Autodesk Fusion 360 part; units mm, degrees
(part 2 of 3)
  spline S21 degree 5 poles (-5.7507, 8.7852) (-5.7508, 8.7791) (-5.7509, 8.7671) (-5.7511, 8.7491) (-5.7512, 8.7251) (-5.7512, 8.6951) (-5.751, 8.6652) (-5.7507, 8.6353) (-5.7502, 8.6055) (-5.7495, 8.5758) (-5.7487, 8.5461) (-5.7478, 8.5165) (-5.7467, 8.4869) (-5.7454, 8.4574) (-5.7439, 8.428) (-5.7423, 8.3986) (-5.7406, 8.3693) (-5.7387, 8.34) (-5.7366, 8.3109) (-5.7343, 8.2817) (-5.7319, 8.2527) (-5.7293, 8.2237) (-5.7266, 8.1948) (-5.7237, 8.166) (-5.7206, 8.1372) (-5.7174, 8.1086) (-5.714, 8.0799) (-5.7104, 8.0514) (-5.7067, 8.023) (-5.7027, 7.9946) (-5.6987, 7.9663) (-5.6944, 7.9381) (-5.69, 7.91) (-5.6854, 7.8819) (-5.6806, 7.854) (-5.6756, 7.8261) (-5.6705, 7.7983) (-5.6652, 7.7706) (-5.6597, 7.743) (-5.654, 7.7156) (-5.6482, 7.6882) (-5.6421, 7.6609) (-5.6359, 7.6337) (-5.6295, 7.6066) (-5.6228, 7.5796) (-5.616, 7.5527) (-5.609, 7.5259) (-5.6019, 7.4993) (-5.5945, 7.4727) (-5.5869, 7.4463) (-5.5791, 7.42) (-5.5711, 7.3938) (-5.5629, 7.3677) (-5.5544, 7.3418) (-5.5457, 7.316) (-5.5368, 7.2904) (-5.5277, 7.2649) (-5.5184, 7.2395) (-5.5089, 7.2142) (-5.4992, 7.1891) (-5.4892, 7.1642) (-5.4788, 7.1395) (-5.4681, 7.115) (-5.4571, 7.0908) (-5.4457, 7.0667) (-5.4342, 7.0428) (-5.4224, 7.0191) (-5.4105, 6.9954) (-5.3984, 6.972) (-5.3859, 6.9488) (-5.3726, 6.9261) (-5.3612, 6.9086) (-5.3521, 6.8957) (-5.3458, 6.8874) (-5.3426, 6.8832) knots -1 -1 -1 -1 -1 -1 -0.98571429 -0.97142857 -0.95714286 -0.94285714 -0.92857143 -0.91428571 -0.9 -0.88571429 -0.87142857 -0.85714286 -0.84285714 -0.82857143 -0.81428571 -0.8 -0.78571429 -0.77142857 -0.75714286 -0.74285714 -0.72857143 -0.71428571 -0.7 -0.68571429 -0.67142857 -0.65714286 -0.64285714 -0.62857143 -0.61428571 -0.6 -0.58571429 -0.57142857 -0.55714286 -0.54285714 -0.52857143 -0.51428571 -0.5 -0.48571429 -0.47142857 -0.45714286 -0.44285714 -0.42857143 -0.41428571 -0.4 -0.38571429 -0.37142857 -0.35714286 -0.34285714 -0.32857143 -0.31428571 -0.3 -0.28571429 -0.27142857 -0.25714286 -0.24285714 -0.22857143 -0.21428571 -0.2 -0.18571429 -0.17142857 -0.15714286 -0.14285714 -0.12857143 -0.11428571 -0.1 -0.08571429 -0.07142857 -0.05714286 -0.04285714 -0.02857143 -0.01428571 0 0 0 0 0 0
  line L21 (-5.3426, 6.8832) -> (-4.7509, 6.121)
  arc A42 (-4.8145, 5.44) -> (-4.7509, 6.121) centre (-5.1459, 5.8144) ccw
  arc A43 (-4.8145, 5.44) -> (-5.44, 4.8145) centre (0, 0) ccw
  arc A44 (-6.121, 4.7509) -> (-5.44, 4.8145) centre (-5.8144, 5.1459) ccw
  line L22 (-6.121, 4.7509) -> (-6.8832, 5.3426)
  spline S22 degree 5 poles (-6.8832, 5.3426) (-6.8874, 5.3458) (-6.8957, 5.3521) (-6.9086, 5.3612) (-6.9261, 5.3726) (-6.9488, 5.3859) (-6.972, 5.3984) (-6.9954, 5.4105) (-7.0191, 5.4224) (-7.0428, 5.4342) (-7.0667, 5.4457) (-7.0908, 5.4571) (-7.115, 5.4681) (-7.1395, 5.4788) (-7.1642, 5.4892) (-7.1891, 5.4992) (-7.2142, 5.5089) (-7.2395, 5.5184) (-7.2649, 5.5277) (-7.2904, 5.5368) (-7.316, 5.5457) (-7.3418, 5.5544) (-7.3677, 5.5629) (-7.3938, 5.5711) (-7.42, 5.5791) (-7.4463, 5.5869) (-7.4727, 5.5945) (-7.4993, 5.6019) (-7.5259, 5.609) (-7.5527, 5.616) (-7.5796, 5.6228) (-7.6066, 5.6295) (-7.6337, 5.6359) (-7.6609, 5.6421) (-7.6882, 5.6482) (-7.7156, 5.654) (-7.743, 5.6597) (-7.7706, 5.6652) (-7.7983, 5.6705) (-7.8261, 5.6756) (-7.854, 5.6806) (-7.8819, 5.6854) (-7.91, 5.69) (-7.9381, 5.6944) (-7.9663, 5.6987) (-7.9946, 5.7027) (-8.023, 5.7067) (-8.0514, 5.7104) (-8.0799, 5.714) (-8.1086, 5.7174) (-8.1372, 5.7206) (-8.166, 5.7237) (-8.1948, 5.7266) (-8.2237, 5.7293) (-8.2527, 5.7319) (-8.2817, 5.7343) (-8.3109, 5.7366) (-8.34, 5.7387) (-8.3693, 5.7406) (-8.3986, 5.7423) (-8.428, 5.7439) (-8.4574, 5.7454) (-8.4869, 5.7467) (-8.5165, 5.7478) (-8.5461, 5.7487) (-8.5758, 5.7495) (-8.6055, 5.7502) (-8.6353, 5.7507) (-8.6652, 5.751) (-8.6951, 5.7512) (-8.7251, 5.7512) (-8.7491, 5.7511) (-8.7671, 5.7509) (-8.7791, 5.7508) (-8.7852, 5.7507) knots 0 0 0 0 0 0 0.01428571 0.02857143 0.04285714 0.05714286 0.07142857 0.08571429 0.1 0.11428571 0.12857143 0.14285714 0.15714286 0.17142857 0.18571429 0.2 0.21428571 0.22857143 0.24285714 0.25714286 0.27142857 0.28571429 0.3 0.31428571 0.32857143 0.34285714 0.35714286 0.37142857 0.38571429 0.4 0.41428571 0.42857143 0.44285714 0.45714286 0.47142857 0.48571429 0.5 0.51428571 0.52857143 0.54285714 0.55714286 0.57142857 0.58571429 0.6 0.61428571 0.62857143 0.64285714 0.65714286 0.67142857 0.68571429 0.7 0.71428571 0.72857143 0.74285714 0.75714286 0.77142857 0.78571429 0.8 0.81428571 0.82857143 0.84285714 0.85714286 0.87142857 0.88571429 0.9 0.91428571 0.92857143 0.94285714 0.95714286 0.97142857 0.98571429 1 1 1 1 1 1
  arc A45 (-8.7852, 5.7507) -> (-9.3729, 4.7328) centre (0, 0) ccw
  spline S23 degree 5 poles (-9.3729, 4.7328) (-9.3699, 4.7276) (-9.364, 4.7171) (-9.3551, 4.7014) (-9.3432, 4.6805) (-9.3282, 4.6546) (-9.3131, 4.6288) (-9.2979, 4.6031) (-9.2826, 4.5775) (-9.2671, 4.5521) (-9.2516, 4.5268) (-9.236, 4.5016) (-9.2202, 4.4766) (-9.2044, 4.4516) (-9.1884, 4.4269) (-9.1723, 4.4022) (-9.1561, 4.3777) (-9.1398, 4.3534) (-9.1234, 4.3291) (-9.1069, 4.305) (-9.0903, 4.2811) (-9.0736, 4.2573) (-9.0568, 4.2336) (-9.0399, 4.2101) (-9.0228, 4.1867) (-9.0057, 4.1635) (-8.9884, 4.1404) (-8.9711, 4.1175) (-8.9536, 4.0948) (-8.936, 4.0721) (-8.9183, 4.0497) (-8.9005, 4.0274) (-8.8826, 4.0052) (-8.8646, 3.9833) (-8.8465, 3.9614) (-8.8283, 3.9398) (-8.8099, 3.9183) (-8.7915, 3.897) (-8.773, 3.8758) (-8.7543, 3.8549) (-8.7355, 3.8341) (-8.7166, 3.8134) (-8.6976, 3.793) (-8.6785, 3.7728) (-8.6593, 3.7527) (-8.64, 3.7328) (-8.6205, 3.7131) (-8.601, 3.6936) (-8.5813, 3.6743) (-8.5615, 3.6552) (-8.5416, 3.6363) (-8.5216, 3.6176) (-8.5014, 3.5992) (-8.4812, 3.581) (-8.4608, 3.563) (-8.4402, 3.5453) (-8.4196, 3.5277) (-8.3989, 3.5104) (-8.378, 3.4932) (-8.357, 3.4764) (-8.3359, 3.4598) (-8.3146, 3.4436) (-8.293, 3.4277) (-8.2714, 3.4122) (-8.2495, 3.3971) (-8.2275, 3.3822) (-8.2055, 3.3675) (-8.1834, 3.3529) (-8.1611, 3.3387) (-8.1387, 3.3249) (-8.1159, 3.3119) (-8.0972, 3.3024) (-8.0829, 3.2958) (-8.0733, 3.2917) (-8.0684, 3.2898) knots -1 -1 -1 -1 -1 -1 -0.98571429 -0.97142857 -0.95714286 -0.94285714 -0.92857143 -0.91428571 -0.9 -0.88571429 -0.87142857 -0.85714286 -0.84285714 -0.82857143 -0.81428571 -0.8 -0.78571429 -0.77142857 -0.75714286 -0.74285714 -0.72857143 -0.71428571 -0.7 -0.68571429 -0.67142857 -0.65714286 -0.64285714 -0.62857143 -0.61428571 -0.6 -0.58571429 -0.57142857 -0.55714286 -0.54285714 -0.52857143 -0.51428571 -0.5 -0.48571429 -0.47142857 -0.45714286 -0.44285714 -0.42857143 -0.41428571 -0.4 -0.38571429 -0.37142857 -0.35714286 -0.34285714 -0.32857143 -0.31428571 -0.3 -0.28571429 -0.27142857 -0.25714286 -0.24285714 -0.22857143 -0.21428571 -0.2 -0.18571429 -0.17142857 -0.15714286 -0.14285714 -0.12857143 -0.11428571 -0.1 -0.08571429 -0.07142857 -0.05714286 -0.04285714 -0.02857143 -0.01428571 0 0 0 0 0 0
  line L23 (-8.0684, 3.2898) -> (-7.1749, 2.9254)
  arc A46 (-6.8895, 2.3039) -> (-7.1749, 2.9254) centre (-7.3637, 2.4624) ccw
  arc A47 (-6.8895, 2.3039) -> (-7.1184, 1.4495) centre (0, 0) ccw
  circle A48 centre (0, 0) radius 1.25
  line L24 (-9.0903, -5.085) -> (-5.33, 8.9489)
  arc A49 (-2.722, 8.2501) -> (-5.33, 8.9489) centre (-4.026, 8.5995) ccw
  line L25 (-2.722, 8.2501) -> (-6.4823, -5.7838)
  arc A50 (-9.0903, -5.085) -> (-6.4823, -5.7838) centre (-7.7863, -5.4344) ccw
  line L26 (-7.7981, 1.2832) -> (-9.4767, -4.9815)
  arc A51 (-9.4767, -4.9815) -> (-6.096, -5.8874) centre (-7.7863, -5.4344) ccw
  line L27 (-6.096, -5.8874) -> (-2.3356, 8.1466)
  arc A52 (-2.3356, 8.1466) -> (-5.7163, 9.0525) centre (-4.026, 8.5995) ccw
  line L28 (-5.7163, 9.0525) -> (-7.2804, 3.2151)
  line L29 (-7.2804, 3.2151) -> (-36.2582, 10.9797)
  line L30 (-36.2582, 10.9797) -> (-36.7759, 9.0478)
  line L31 (-36.7759, 9.0478) -> (-7.7981, 1.2832)
  circle A53 centre (-5.8457, 1.7953) radius 1.15
extrude "Extrude1" add sketch "sketch 238" along normal blind 2 contours A0 L0 S23 L23 A46 L24 L26 L29 L30 L31 | A0 L0 L1 L24 L26 | L1 S2 A5 L3 A6 L24 L25 A50 L26 A51 L27 | L22 S23 L23 A46 L24 L28 L29 | S2 A5 L24 A50 | A40 L20 A41 S21 L22 L24 A49 L25 L27 A52 L28 | A41 S21 L24 A49 | L3 A6 A40 L20 L25 L27
sketch "Sketch1" plane through (0, 0, 5) normal (0, 0, 1) x (-1, 0, 0)
  arc A0 (-2.722, 8.2501) -> (-5.33, 8.9489) centre (-4.026, 8.5995) ccw
  line L0 (-2.722, 8.2501) -> (-6.4823, -5.7838)
  arc A1 (-9.0903, -5.085) -> (-6.4823, -5.7838) centre (-7.7863, -5.4344) ccw
  line L1 (-9.0903, -5.085) -> (-5.33, 8.9489)
  line L2 (-36.7759, 9.0478) -> (-7.7981, 1.2832)
  line L3 (-7.7981, 1.2832) -> (-9.4767, -4.9815)
  arc A2 (-9.4767, -4.9815) -> (-6.096, -5.8874) centre (-7.7863, -5.4344) ccw
  line L4 (-6.096, -5.8874) -> (-2.3356, 8.1466)
  arc A3 (-2.3356, 8.1466) -> (-5.7163, 9.0525) centre (-4.026, 8.5995) ccw
  line L5 (-5.7163, 9.0525) -> (-7.2804, 3.2151)
  line L6 (-7.2804, 3.2151) -> (-36.2582, 10.9797)
  line L7 (-36.2582, 10.9797) -> (-36.7759, 9.0478)
  line L8 (-4.6022, 1.2331) -> (-7.2102, 1.932)
  line L9 (-7.2102, 1.932) -> (-7.214, 1.933)
  line L10 (-6.9513, 2.8979) -> (-36.2582, 10.9797)
  line L11 (-7.2804, 3.2151) -> (-6.8941, 3.1116)
  line L12 (-6.8941, 3.1116) -> (-7.476, 0.9679)
  line L13 (-7.8546, 1.0723) -> (-7.2804, 3.2151)
  line L14 (-7.2804, 3.2151) -> (-36.2582, 10.9797)
  line L15 (-36.2582, 10.9797) -> (-36.7759, 9.0478)
  line L16 (-7.7981, 1.2832) -> (-36.7759, 9.0478)
  line L17 (-7.8546, 1.0723) -> (-36.7759, 9.0478)
  point P0 (-7.3369, 3.0042)
  constraint midpoint L0 L8.start
  constraint midpoint L1 L8.end
  constraint coincident L1 L10.start
  constraint coincident L5.end L6.start
  constraint coincident L1 L11.end
  constraint perpendicular L1 L11
  constraint coincident L3 L13.start
  constraint coincident L6.end L7.start
  constraint coincident L2.start L7.end
  constraint coincident L2.end L3.start
  constraint coincident L13 P0
  constraint coincident L10 P0
extrude "Extrude2" cut sketch "Sketch1" against normal blind 9.5 contours L6 L10 L13 L14
extrude "Extrude3" add sketch "Sketch1" against normal blind 2 contours L2 L3 L13 L16 L17

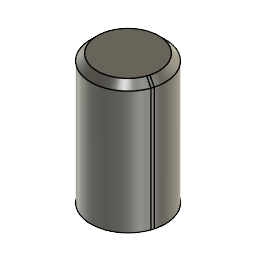
design "MiniKey_GearPin"
Autodesk Fusion 360 part; units mm, degrees
other "Sketch1"
sketch "sketch 232" plane through (0, 0, 3) normal (0, 0, 1) x (-1, 0, 0)
  arc A0 (-7.6764, 1.0539) -> (-7.1184, 1.4495) centre (-7.6084, 1.5493) ccw
  line L0 (-7.6764, 1.0539) -> (-8.6323, 1.1852)
  spline S0 degree 5 poles (-8.6323, 1.1852) (-8.6375, 1.1859) (-8.6479, 1.1872) (-8.6636, 1.1886) (-8.6845, 1.1897) (-8.7108, 1.1899) (-8.7371, 1.1892) (-8.7635, 1.188) (-8.7899, 1.1864) (-8.8164, 1.1847) (-8.8428, 1.1828) (-8.8693, 1.1806) (-8.8958, 1.178) (-8.9224, 1.1751) (-8.949, 1.1717) (-8.9756, 1.1679) (-9.0022, 1.1638) (-9.0288, 1.1594) (-9.0554, 1.1547) (-9.0821, 1.1498) (-9.1087, 1.1447) (-9.1354, 1.1393) (-9.1621, 1.1337) (-9.1887, 1.1278) (-9.2154, 1.1217) (-9.2421, 1.1153) (-9.2688, 1.1086) (-9.2955, 1.1017) (-9.3222, 1.0946) (-9.3488, 1.0873) (-9.3755, 1.0797) (-9.4022, 1.072) (-9.4289, 1.064) (-9.4555, 1.0558) (-9.4822, 1.0474) (-9.5089, 1.0387) (-9.5355, 1.0299) (-9.5622, 1.0209) (-9.5888, 1.0116) (-9.6154, 1.0022) (-9.642, 0.9925) (-9.6686, 0.9827) (-9.6952, 0.9727) (-9.7218, 0.9624) (-9.7483, 0.952) (-9.7749, 0.9414) (-9.8014, 0.9306) (-9.8279, 0.9196) (-9.8544, 0.9085) (-9.8809, 0.8971) (-9.9074, 0.8856) (-9.9338, 0.8739) (-9.9602, 0.862) (-9.9866, 0.8499) (-10.013, 0.8376) (-10.0394, 0.8252) (-10.0657, 0.8126) (-10.092, 0.7998) (-10.1183, 0.7868) (-10.1446, 0.7737) (-10.1708, 0.7604) (-10.197, 0.7469) (-10.2232, 0.7333) (-10.2494, 0.7195) (-10.2755, 0.7055) (-10.3016, 0.6914) (-10.3277, 0.677) (-10.3538, 0.6626) (-10.3798, 0.6479) (-10.4058, 0.6331) (-10.4317, 0.6182) (-10.4525, 0.6061) (-10.468, 0.5969) (-10.4784, 0.5908) (-10.4835, 0.5877) knots 0 0 0 0 0 0 0.01428571 0.02857143 0.04285714 0.05714286 0.07142857 0.08571429 0.1 0.11428571 0.12857143 0.14285714 0.15714286 0.17142857 0.18571429 0.2 0.21428571 0.22857143 0.24285714 0.25714286 0.27142857 0.28571429 0.3 0.31428571 0.32857143 0.34285714 0.35714286 0.37142857 0.38571429 0.4 0.41428571 0.42857143 0.44285714 0.45714286 0.47142857 0.48571429 0.5 0.51428571 0.52857143 0.54285714 0.55714286 0.57142857 0.58571429 0.6 0.61428571 0.62857143 0.64285714 0.65714286 0.67142857 0.68571429 0.7 0.71428571 0.72857143 0.74285714 0.75714286 0.77142857 0.78571429 0.8 0.81428571 0.82857143 0.84285714 0.85714286 0.87142857 0.88571429 0.9 0.91428571 0.92857143 0.94285714 0.95714286 0.97142857 0.98571429 1 1 1 1 1 1
  arc A1 (-10.4835, 0.5877) -> (-10.4835, -0.5877) centre (0, 0) ccw
  spline S1 degree 5 poles (-10.4835, -0.5877) (-10.4784, -0.5908) (-10.468, -0.5969) (-10.4525, -0.6061) (-10.4317, -0.6182) (-10.4058, -0.6331) (-10.3798, -0.6479) (-10.3538, -0.6626) (-10.3277, -0.677) (-10.3016, -0.6914) (-10.2755, -0.7055) (-10.2494, -0.7195) (-10.2232, -0.7333) (-10.197, -0.7469) (-10.1708, -0.7604) (-10.1446, -0.7737) (-10.1183, -0.7868) (-10.092, -0.7998) (-10.0657, -0.8126) (-10.0394, -0.8252) (-10.013, -0.8376) (-9.9866, -0.8499) (-9.9602, -0.862) (-9.9338, -0.8739) (-9.9074, -0.8856) (-9.8809, -0.8971) (-9.8544, -0.9085) (-9.8279, -0.9196) (-9.8014, -0.9306) (-9.7749, -0.9414) (-9.7483, -0.952) (-9.7218, -0.9624) (-9.6952, -0.9727) (-9.6686, -0.9827) (-9.642, -0.9925) (-9.6154, -1.0022) (-9.5888, -1.0116) (-9.5622, -1.0209) (-9.5355, -1.0299) (-9.5089, -1.0387) (-9.4822, -1.0474) (-9.4555, -1.0558) (-9.4289, -1.064) (-9.4022, -1.072) (-9.3755, -1.0797) (-9.3488, -1.0873) (-9.3222, -1.0946) (-9.2955, -1.1017) (-9.2688, -1.1086) (-9.2421, -1.1153) (-9.2154, -1.1217) (-9.1887, -1.1278) (-9.1621, -1.1337) (-9.1354, -1.1393) (-9.1087, -1.1447) (-9.0821, -1.1498) (-9.0554, -1.1547) (-9.0288, -1.1594) (-9.0022, -1.1638) (-8.9756, -1.1679) (-8.949, -1.1717) (-8.9224, -1.1751) (-8.8958, -1.178) (-8.8693, -1.1806) (-8.8428, -1.1828) (-8.8164, -1.1847) (-8.7899, -1.1864) (-8.7635, -1.188) (-8.7371, -1.1892) (-8.7108, -1.1899) (-8.6845, -1.1897) (-8.6636, -1.1886) (-8.6479, -1.1872) (-8.6375, -1.1859) (-8.6323, -1.1852) knots -1 -1 -1 -1 -1 -1 -0.98571429 -0.97142857 -0.95714286 -0.94285714 -0.92857143 -0.91428571 -0.9 -0.88571429 -0.87142857 -0.85714286 -0.84285714 -0.82857143 -0.81428571 -0.8 -0.78571429 -0.77142857 -0.75714286 -0.74285714 -0.72857143 -0.71428571 -0.7 -0.68571429 -0.67142857 -0.65714286 -0.64285714 -0.62857143 -0.61428571 -0.6 -0.58571429 -0.57142857 -0.55714286 -0.54285714 -0.52857143 -0.51428571 -0.5 -0.48571429 -0.47142857 -0.45714286 -0.44285714 -0.42857143 -0.41428571 -0.4 -0.38571429 -0.37142857 -0.35714286 -0.34285714 -0.32857143 -0.31428571 -0.3 -0.28571429 -0.27142857 -0.25714286 -0.24285714 -0.22857143 -0.21428571 -0.2 -0.18571429 -0.17142857 -0.15714286 -0.14285714 -0.12857143 -0.11428571 -0.1 -0.08571429 -0.07142857 -0.05714286 -0.04285714 -0.02857143 -0.01428571 0 0 0 0 0 0
  line L1 (-8.6323, -1.1852) -> (-7.6764, -1.0539)
  arc A2 (-7.1184, -1.4495) -> (-7.6764, -1.0539) centre (-7.6084, -1.5493) ccw
  arc A3 (-7.1184, -1.4495) -> (-6.8895, -2.3039) centre (0, 0) ccw
  arc A4 (-7.1749, -2.9254) -> (-6.8895, -2.3039) centre (-7.3637, -2.4624) ccw
  line L2 (-7.1749, -2.9254) -> (-8.0684, -3.2898)
  spline S2 degree 5 poles (-8.0684, -3.2898) (-8.0733, -3.2917) (-8.0829, -3.2958) (-8.0972, -3.3024) (-8.1159, -3.3119) (-8.1387, -3.3249) (-8.1611, -3.3387) (-8.1834, -3.3529) (-8.2055, -3.3675) (-8.2275, -3.3822) (-8.2495, -3.3971) (-8.2714, -3.4122) (-8.293, -3.4277) (-8.3146, -3.4436) (-8.3359, -3.4598) (-8.357, -3.4764) (-8.378, -3.4932) (-8.3989, -3.5104) (-8.4196, -3.5277) (-8.4402, -3.5453) (-8.4608, -3.563) (-8.4812, -3.581) (-8.5014, -3.5992) (-8.5216, -3.6176) (-8.5416, -3.6363) (-8.5615, -3.6552) (-8.5813, -3.6743) (-8.601, -3.6936) (-8.6205, -3.7131) (-8.64, -3.7328) (-8.6593, -3.7527) (-8.6785, -3.7728) (-8.6976, -3.793) (-8.7166, -3.8134) (-8.7355, -3.8341) (-8.7543, -3.8549) (-8.773, -3.8758) (-8.7915, -3.897) (-8.8099, -3.9183) (-8.8283, -3.9398) (-8.8465, -3.9614) (-8.8646, -3.9833) (-8.8826, -4.0052) (-8.9005, -4.0274) (-8.9183, -4.0497) (-8.936, -4.0721) (-8.9536, -4.0948) (-8.9711, -4.1175) (-8.9884, -4.1404) (-9.0057, -4.1635) (-9.0228, -4.1867) (-9.0399, -4.2101) (-9.0568, -4.2336) (-9.0736, -4.2573) (-9.0903, -4.2811) (-9.1069, -4.305) (-9.1234, -4.3291) (-9.1398, -4.3534) (-9.1561, -4.3777) (-9.1723, -4.4022) (-9.1884, -4.4269) (-9.2044, -4.4516) (-9.2202, -4.4766) (-9.236, -4.5016) (-9.2516, -4.5268) (-9.2671, -4.5521) (-9.2826, -4.5775) (-9.2979, -4.6031) (-9.3131, -4.6288) (-9.3282, -4.6546) (-9.3432, -4.6805) (-9.3551, -4.7014) (-9.364, -4.7171) (-9.3699, -4.7276) (-9.3729, -4.7328) knots 0 0 0 0 0 0 0.01428571 0.02857143 0.04285714 0.05714286 0.07142857 0.08571429 0.1 0.11428571 0.12857143 0.14285714 0.15714286 0.17142857 0.18571429 0.2 0.21428571 0.22857143 0.24285714 0.25714286 0.27142857 0.28571429 0.3 0.31428571 0.32857143 0.34285714 0.35714286 0.37142857 0.38571429 0.4 0.41428571 0.42857143 0.44285714 0.45714286 0.47142857 0.48571429 0.5 0.51428571 0.52857143 0.54285714 0.55714286 0.57142857 0.58571429 0.6 0.61428571 0.62857143 0.64285714 0.65714286 0.67142857 0.68571429 0.7 0.71428571 0.72857143 0.74285714 0.75714286 0.77142857 0.78571429 0.8 0.81428571 0.82857143 0.84285714 0.85714286 0.87142857 0.88571429 0.9 0.91428571 0.92857143 0.94285714 0.95714286 0.97142857 0.98571429 1 1 1 1 1 1
  arc A5 (-9.3729, -4.7328) -> (-8.7852, -5.7507) centre (0, 0) ccw
  spline S3 degree 5 poles (-8.7852, -5.7507) (-8.7791, -5.7508) (-8.7671, -5.7509) (-8.7491, -5.7511) (-8.7251, -5.7512) (-8.6951, -5.7512) (-8.6652, -5.751) (-8.6353, -5.7507) (-8.6055, -5.7502) (-8.5758, -5.7495) (-8.5461, -5.7487) (-8.5165, -5.7478) (-8.4869, -5.7467) (-8.4574, -5.7454) (-8.428, -5.7439) (-8.3986, -5.7423) (-8.3693, -5.7406) (-8.34, -5.7387) (-8.3109, -5.7366) (-8.2817, -5.7343) (-8.2527, -5.7319) (-8.2237, -5.7293) (-8.1948, -5.7266) (-8.166, -5.7237) (-8.1372, -5.7206) (-8.1086, -5.7174) (-8.0799, -5.714) (-8.0514, -5.7104) (-8.023, -5.7067) (-7.9946, -5.7027) (-7.9663, -5.6987) (-7.9381, -5.6944) (-7.91, -5.69) (-7.8819, -5.6854) (-7.854, -5.6806) (-7.8261, -5.6756) (-7.7983, -5.6705) (-7.7706, -5.6652) (-7.743, -5.6597) (-7.7156, -5.654) (-7.6882, -5.6482) (-7.6609, -5.6421) (-7.6337, -5.6359) (-7.6066, -5.6295) (-7.5796, -5.6228) (-7.5527, -5.616) (-7.5259, -5.609) (-7.4993, -5.6019) (-7.4727, -5.5945) (-7.4463, -5.5869) (-7.42, -5.5791) (-7.3938, -5.5711) (-7.3677, -5.5629) (-7.3418, -5.5544) (-7.316, -5.5457) (-7.2904, -5.5368) (-7.2649, -5.5277) (-7.2395, -5.5184) (-7.2142, -5.5089) (-7.1891, -5.4992) (-7.1642, -5.4892) (-7.1395, -5.4788) (-7.115, -5.4681) (-7.0908, -5.4571) (-7.0667, -5.4457) (-7.0428, -5.4342) (-7.0191, -5.4224) (-6.9954, -5.4105) (-6.972, -5.3984) (-6.9488, -5.3859) (-6.9261, -5.3726) (-6.9086, -5.3612) (-6.8957, -5.3521) (-6.8874, -5.3458) (-6.8832, -5.3426) knots -1 -1 -1 -1 -1 -1 -0.98571429 -0.97142857 -0.95714286 -0.94285714 -0.92857143 -0.91428571 -0.9 -0.88571429 -0.87142857 -0.85714286 -0.84285714 -0.82857143 -0.81428571 -0.8 -0.78571429 -0.77142857 -0.75714286 -0.74285714 -0.72857143 -0.71428571 -0.7 -0.68571429 -0.67142857 -0.65714286 -0.64285714 -0.62857143 -0.61428571 -0.6 -0.58571429 -0.57142857 -0.55714286 -0.54285714 -0.52857143 -0.51428571 -0.5 -0.48571429 -0.47142857 -0.45714286 -0.44285714 -0.42857143 -0.41428571 -0.4 -0.38571429 -0.37142857 -0.35714286 -0.34285714 -0.32857143 -0.31428571 -0.3 -0.28571429 -0.27142857 -0.25714286 -0.24285714 -0.22857143 -0.21428571 -0.2 -0.18571429 -0.17142857 -0.15714286 -0.14285714 -0.12857143 -0.11428571 -0.1 -0.08571429 -0.07142857 -0.05714286 -0.04285714 -0.02857143 -0.01428571 0 0 0 0 0 0
  line L3 (-6.8832, -5.3426) -> (-6.121, -4.7509)
  arc A6 (-5.44, -4.8145) -> (-6.121, -4.7509) centre (-5.8144, -5.1459) ccw
  arc A7 (-5.44, -4.8145) -> (-4.8145, -5.44) centre (0, 0) ccw
  arc A8 (-4.7509, -6.121) -> (-4.8145, -5.44) centre (-5.1459, -5.8144) ccw
  line L4 (-4.7509, -6.121) -> (-5.3426, -6.8832)
  spline S4 degree 5 poles (-5.3426, -6.8832) (-5.3458, -6.8874) (-5.3521, -6.8957) (-5.3612, -6.9086) (-5.3726, -6.9261) (-5.3859, -6.9488) (-5.3984, -6.972) (-5.4105, -6.9954) (-5.4224, -7.0191) (-5.4342, -7.0428) (-5.4457, -7.0667) (-5.4571, -7.0908) (-5.4681, -7.115) (-5.4788, -7.1395) (-5.4892, -7.1642) (-5.4992, -7.1891) (-5.5089, -7.2142) (-5.5184, -7.2395) (-5.5277, -7.2649) (-5.5368, -7.2904) (-5.5457, -7.316) (-5.5544, -7.3418) (-5.5629, -7.3677) (-5.5711, -7.3938) (-5.5791, -7.42) (-5.5869, -7.4463) (-5.5945, -7.4727) (-5.6019, -7.4993) (-5.609, -7.5259) (-5.616, -7.5527) (-5.6228, -7.5796) (-5.6295, -7.6066) (-5.6359, -7.6337) (-5.6421, -7.6609) (-5.6482, -7.6882) (-5.654, -7.7156) (-5.6597, -7.743) (-5.6652, -7.7706) (-5.6705, -7.7983) (-5.6756, -7.8261) (-5.6806, -7.854) (-5.6854, -7.8819) (-5.69, -7.91) (-5.6944, -7.9381) (-5.6987, -7.9663) (-5.7027, -7.9946) (-5.7067, -8.023) (-5.7104, -8.0514) (-5.714, -8.0799) (-5.7174, -8.1086) (-5.7206, -8.1372) (-5.7237, -8.166) (-5.7266, -8.1948) (-5.7293, -8.2237) (-5.7319, -8.2527) (-5.7343, -8.2817) (-5.7366, -8.3109) (-5.7387, -8.34) (-5.7406, -8.3693) (-5.7423, -8.3986) (-5.7439, -8.428) (-5.7454, -8.4574) (-5.7467, -8.4869) (-5.7478, -8.5165) (-5.7487, -8.5461) (-5.7495, -8.5758) (-5.7502, -8.6055) (-5.7507, -8.6353) (-5.751, -8.6652) (-5.7512, -8.6951) (-5.7512, -8.7251) (-5.7511, -8.7491) (-5.7509, -8.7671) (-5.7508, -8.7791) (-5.7507, -8.7852) knots 0 0 0 0 0 0 0.01428571 0.02857143 0.04285714 0.05714286 0.07142857 0.08571429 0.1 0.11428571 0.12857143 0.14285714 0.15714286 0.17142857 0.18571429 0.2 0.21428571 0.22857143 0.24285714 0.25714286 0.27142857 0.28571429 0.3 0.31428571 0.32857143 0.34285714 0.35714286 0.37142857 0.38571429 0.4 0.41428571 0.42857143 0.44285714 0.45714286 0.47142857 0.48571429 0.5 0.51428571 0.52857143 0.54285714 0.55714286 0.57142857 0.58571429 0.6 0.61428571 0.62857143 0.64285714 0.65714286 0.67142857 0.68571429 0.7 0.71428571 0.72857143 0.74285714 0.75714286 0.77142857 0.78571429 0.8 0.81428571 0.82857143 0.84285714 0.85714286 0.87142857 0.88571429 0.9 0.91428571 0.92857143 0.94285714 0.95714286 0.97142857 0.98571429 1 1 1 1 1 1
  arc A9 (-5.7507, -8.7852) -> (-4.7328, -9.3729) centre (0, 0) ccw
  spline S5 degree 5 poles (-4.7328, -9.3729) (-4.7276, -9.3699) (-4.7171, -9.364) (-4.7014, -9.3551) (-4.6805, -9.3432) (-4.6546, -9.3282) (-4.6288, -9.3131) (-4.6031, -9.2979) (-4.5775, -9.2826) (-4.5521, -9.2671) (-4.5268, -9.2516) (-4.5016, -9.236) (-4.4766, -9.2202) (-4.4516, -9.2044) (-4.4269, -9.1884) (-4.4022, -9.1723) (-4.3777, -9.1561) (-4.3534, -9.1398) (-4.3291, -9.1234) (-4.305, -9.1069) (-4.2811, -9.0903) (-4.2573, -9.0736) (-4.2336, -9.0568) (-4.2101, -9.0399) (-4.1867, -9.0228) (-4.1635, -9.0057) (-4.1404, -8.9884) (-4.1175, -8.9711) (-4.0948, -8.9536) (-4.0721, -8.936) (-4.0497, -8.9183) (-4.0274, -8.9005) (-4.0052, -8.8826) (-3.9833, -8.8646) (-3.9614, -8.8465) (-3.9398, -8.8283) (-3.9183, -8.8099) (-3.897, -8.7915) (-3.8758, -8.773) (-3.8549, -8.7543) (-3.8341, -8.7355) (-3.8134, -8.7166) (-3.793, -8.6976) (-3.7728, -8.6785) (-3.7527, -8.6593) (-3.7328, -8.64) (-3.7131, -8.6205) (-3.6936, -8.601) (-3.6743, -8.5813) (-3.6552, -8.5615) (-3.6363, -8.5416) (-3.6176, -8.5216) (-3.5992, -8.5014) (-3.581, -8.4812) (-3.563, -8.4608) (-3.5453, -8.4402) (-3.5277, -8.4196) (-3.5104, -8.3989) (-3.4932, -8.378) (-3.4764, -8.357) (-3.4598, -8.3359) (-3.4436, -8.3146) (-3.4277, -8.293) (-3.4122, -8.2714) (-3.3971, -8.2495) (-3.3822, -8.2275) (-3.3675, -8.2055) (-3.3529, -8.1834) (-3.3387, -8.1611) (-3.3249, -8.1387) (-3.3119, -8.1159) (-3.3024, -8.0972) (-3.2958, -8.0829) (-3.2917, -8.0733) (-3.2898, -8.0684) knots -1 -1 -1 -1 -1 -1 -0.98571429 -0.97142857 -0.95714286 -0.94285714 -0.92857143 -0.91428571 -0.9 -0.88571429 -0.87142857 -0.85714286 -0.84285714 -0.82857143 -0.81428571 -0.8 -0.78571429 -0.77142857 -0.75714286 -0.74285714 -0.72857143 -0.71428571 -0.7 -0.68571429 -0.67142857 -0.65714286 -0.64285714 -0.62857143 -0.61428571 -0.6 -0.58571429 -0.57142857 -0.55714286 -0.54285714 -0.52857143 -0.51428571 -0.5 -0.48571429 -0.47142857 -0.45714286 -0.44285714 -0.42857143 -0.41428571 -0.4 -0.38571429 -0.37142857 -0.35714286 -0.34285714 -0.32857143 -0.31428571 -0.3 -0.28571429 -0.27142857 -0.25714286 -0.24285714 -0.22857143 -0.21428571 -0.2 -0.18571429 -0.17142857 -0.15714286 -0.14285714 -0.12857143 -0.11428571 -0.1 -0.08571429 -0.07142857 -0.05714286 -0.04285714 -0.02857143 -0.01428571 0 0 0 0 0 0
  line L5 (-3.2898, -8.0684) -> (-2.9254, -7.1749)
  arc A10 (-2.3039, -6.8895) -> (-2.9254, -7.1749) centre (-2.4624, -7.3637) ccw
  arc A11 (-2.3039, -6.8895) -> (-1.4495, -7.1184) centre (0, 0) ccw
  arc A12 (-1.0539, -7.6764) -> (-1.4495, -7.1184) centre (-1.5493, -7.6084) ccw
  line L6 (-1.0539, -7.6764) -> (-1.1852, -8.6323)
  spline S6 degree 5 poles (-1.1852, -8.6323) (-1.1859, -8.6375) (-1.1872, -8.6479) (-1.1886, -8.6636) (-1.1897, -8.6845) (-1.1899, -8.7108) (-1.1892, -8.7371) (-1.188, -8.7635) (-1.1864, -8.7899) (-1.1847, -8.8164) (-1.1828, -8.8428) (-1.1806, -8.8693) (-1.178, -8.8958) (-1.1751, -8.9224) (-1.1717, -8.949) (-1.1679, -8.9756) (-1.1638, -9.0022) (-1.1594, -9.0288) (-1.1547, -9.0554) (-1.1498, -9.0821) (-1.1447, -9.1087) (-1.1393, -9.1354) (-1.1337, -9.1621) (-1.1278, -9.1887) (-1.1217, -9.2154) (-1.1153, -9.2421) (-1.1086, -9.2688) (-1.1017, -9.2955) (-1.0946, -9.3222) (-1.0873, -9.3488) (-1.0797, -9.3755) (-1.072, -9.4022) (-1.064, -9.4289) (-1.0558, -9.4555) (-1.0474, -9.4822) (-1.0387, -9.5089) (-1.0299, -9.5355) (-1.0209, -9.5622) (-1.0116, -9.5888) (-1.0022, -9.6154) (-0.9925, -9.642) (-0.9827, -9.6686) (-0.9727, -9.6952) (-0.9624, -9.7218) (-0.952, -9.7483) (-0.9414, -9.7749) (-0.9306, -9.8014) (-0.9196, -9.8279) (-0.9085, -9.8544) (-0.8971, -9.8809) (-0.8856, -9.9074) (-0.8739, -9.9338) (-0.862, -9.9602) (-0.8499, -9.9866) (-0.8376, -10.013) (-0.8252, -10.0394) (-0.8126, -10.0657) (-0.7998, -10.092) (-0.7868, -10.1183) (-0.7737, -10.1446) (-0.7604, -10.1708) (-0.7469, -10.197) (-0.7333, -10.2232) (-0.7195, -10.2494) (-0.7055, -10.2755) (-0.6914, -10.3016) (-0.677, -10.3277) (-0.6626, -10.3538) (-0.6479, -10.3798) (-0.6331, -10.4058) (-0.6182, -10.4317) (-0.6061, -10.4525) (-0.5969, -10.468) (-0.5908, -10.4784) (-0.5877, -10.4835) knots 0 0 0 0 0 0 0.01428571 0.02857143 0.04285714 0.05714286 0.07142857 0.08571429 0.1 0.11428571 0.12857143 0.14285714 0.15714286 0.17142857 0.18571429 0.2 0.21428571 0.22857143 0.24285714 0.25714286 0.27142857 0.28571429 0.3 0.31428571 0.32857143 0.34285714 0.35714286 0.37142857 0.38571429 0.4 0.41428571 0.42857143 0.44285714 0.45714286 0.47142857 0.48571429 0.5 0.51428571 0.52857143 0.54285714 0.55714286 0.57142857 0.58571429 0.6 0.61428571 0.62857143 0.64285714 0.65714286 0.67142857 0.68571429 0.7 0.71428571 0.72857143 0.74285714 0.75714286 0.77142857 0.78571429 0.8 0.81428571 0.82857143 0.84285714 0.85714286 0.87142857 0.88571429 0.9 0.91428571 0.92857143 0.94285714 0.95714286 0.97142857 0.98571429 1 1 1 1 1 1
  arc A13 (-0.5877, -10.4835) -> (0.5877, -10.4835) centre (0, 0) ccw
  spline S7 degree 5 poles (0.5877, -10.4835) (0.5908, -10.4784) (0.5969, -10.468) (0.6061, -10.4525) (0.6182, -10.4317) (0.6331, -10.4058) (0.6479, -10.3798) (0.6626, -10.3538) (0.677, -10.3277) (0.6914, -10.3016) (0.7055, -10.2755) (0.7195, -10.2494) (0.7333, -10.2232) (0.7469, -10.197) (0.7604, -10.1708) (0.7737, -10.1446) (0.7868, -10.1183) (0.7998, -10.092) (0.8126, -10.0657) (0.8252, -10.0394) (0.8376, -10.013) (0.8499, -9.9866) (0.862, -9.9602) (0.8739, -9.9338) (0.8856, -9.9074) (0.8971, -9.8809) (0.9085, -9.8544) (0.9196, -9.8279) (0.9306, -9.8014) (0.9414, -9.7749) (0.952, -9.7483) (0.9624, -9.7218) (0.9727, -9.6952) (0.9827, -9.6686) (0.9925, -9.642) (1.0022, -9.6154) (1.0116, -9.5888) (1.0209, -9.5622) (1.0299, -9.5355) (1.0387, -9.5089) (1.0474, -9.4822) (1.0558, -9.4555) (1.064, -9.4289) (1.072, -9.4022) (1.0797, -9.3755) (1.0873, -9.3488) (1.0946, -9.3222) (1.1017, -9.2955) (1.1086, -9.2688) (1.1153, -9.2421) (1.1217, -9.2154) (1.1278, -9.1887) (1.1337, -9.1621) (1.1393, -9.1354) (1.1447, -9.1087) (1.1498, -9.0821) (1.1547, -9.0554) (1.1594, -9.0288) (1.1638, -9.0022) (1.1679, -8.9756) (1.1717, -8.949) (1.1751, -8.9224) (1.178, -8.8958) (1.1806, -8.8693) (1.1828, -8.8428) (1.1847, -8.8164) (1.1864, -8.7899) (1.188, -8.7635) (1.1892, -8.7371) (1.1899, -8.7108) (1.1897, -8.6845) (1.1886, -8.6636) (1.1872, -8.6479) (1.1859, -8.6375) (1.1852, -8.6323) knots -1 -1 -1 -1 -1 -1 -0.98571429 -0.97142857 -0.95714286 -0.94285714 -0.92857143 -0.91428571 -0.9 -0.88571429 -0.87142857 -0.85714286 -0.84285714 -0.82857143 -0.81428571 -0.8 -0.78571429 -0.77142857 -0.75714286 -0.74285714 -0.72857143 -0.71428571 -0.7 -0.68571429 -0.67142857 -0.65714286 -0.64285714 -0.62857143 -0.61428571 -0.6 -0.58571429 -0.57142857 -0.55714286 -0.54285714 -0.52857143 -0.51428571 -0.5 -0.48571429 -0.47142857 -0.45714286 -0.44285714 -0.42857143 -0.41428571 -0.4 -0.38571429 -0.37142857 -0.35714286 -0.34285714 -0.32857143 -0.31428571 -0.3 -0.28571429 -0.27142857 -0.25714286 -0.24285714 -0.22857143 -0.21428571 -0.2 -0.18571429 -0.17142857 -0.15714286 -0.14285714 -0.12857143 -0.11428571 -0.1 -0.08571429 -0.07142857 -0.05714286 -0.04285714 -0.02857143 -0.01428571 0 0 0 0 0 0
  line L7 (1.1852, -8.6323) -> (1.0539, -7.6764)
  arc A14 (1.4495, -7.1184) -> (1.0539, -7.6764) centre (1.5493, -7.6084) ccw
  arc A15 (1.4495, -7.1184) -> (2.3039, -6.8895) centre (0, 0) ccw
  arc A16 (2.9254, -7.1749) -> (2.3039, -6.8895) centre (2.4624, -7.3637) ccw
  line L8 (2.9254, -7.1749) -> (3.2898, -8.0684)
  spline S8 degree 5 poles (3.2898, -8.0684) (3.2917, -8.0733) (3.2958, -8.0829) (3.3024, -8.0972) (3.3119, -8.1159) (3.3249, -8.1387) (3.3387, -8.1611) (3.3529, -8.1834) (3.3675, -8.2055) (3.3822, -8.2275) (3.3971, -8.2495) (3.4122, -8.2714) (3.4277, -8.293) (3.4436, -8.3146) (3.4598, -8.3359) (3.4764, -8.357) (3.4932, -8.378) (3.5104, -8.3989) (3.5277, -8.4196) (3.5453, -8.4402) (3.563, -8.4608) (3.581, -8.4812) (3.5992, -8.5014) (3.6176, -8.5216) (3.6363, -8.5416) (3.6552, -8.5615) (3.6743, -8.5813) (3.6936, -8.601) (3.7131, -8.6205) (3.7328, -8.64) (3.7527, -8.6593) (3.7728, -8.6785) (3.793, -8.6976) (3.8134, -8.7166) (3.8341, -8.7355) (3.8549, -8.7543) (3.8758, -8.773) (3.897, -8.7915) (3.9183, -8.8099) (3.9398, -8.8283) (3.9614, -8.8465) (3.9833, -8.8646) (4.0052, -8.8826) (4.0274, -8.9005) (4.0497, -8.9183) (4.0721, -8.936) (4.0948, -8.9536) (4.1175, -8.9711) (4.1404, -8.9884) (4.1635, -9.0057) (4.1867, -9.0228) (4.2101, -9.0399) (4.2336, -9.0568) (4.2573, -9.0736) (4.2811, -9.0903) (4.305, -9.1069) (4.3291, -9.1234) (4.3534, -9.1398) (4.3777, -9.1561) (4.4022, -9.1723) (4.4269, -9.1884) (4.4516, -9.2044) (4.4766, -9.2202) (4.5016, -9.236) (4.5268, -9.2516) (4.5521, -9.2671) (4.5775, -9.2826) (4.6031, -9.2979) (4.6288, -9.3131) (4.6546, -9.3282) (4.6805, -9.3432) (4.7014, -9.3551) (4.7171, -9.364) (4.7276, -9.3699) (4.7328, -9.3729) knots 0 0 0 0 0 0 0.01428571 0.02857143 0.04285714 0.05714286 0.07142857 0.08571429 0.1 0.11428571 0.12857143 0.14285714 0.15714286 0.17142857 0.18571429 0.2 0.21428571 0.22857143 0.24285714 0.25714286 0.27142857 0.28571429 0.3 0.31428571 0.32857143 0.34285714 0.35714286 0.37142857 0.38571429 0.4 0.41428571 0.42857143 0.44285714 0.45714286 0.47142857 0.48571429 0.5 0.51428571 0.52857143 0.54285714 0.55714286 0.57142857 0.58571429 0.6 0.61428571 0.62857143 0.64285714 0.65714286 0.67142857 0.68571429 0.7 0.71428571 0.72857143 0.74285714 0.75714286 0.77142857 0.78571429 0.8 0.81428571 0.82857143 0.84285714 0.85714286 0.87142857 0.88571429 0.9 0.91428571 0.92857143 0.94285714 0.95714286 0.97142857 0.98571429 1 1 1 1 1 1
  arc A17 (4.7328, -9.3729) -> (5.7507, -8.7852) centre (0, 0) ccw
  spline S9 degree 5 poles (5.7507, -8.7852) (5.7508, -8.7791) (5.7509, -8.7671) (5.7511, -8.7491) (5.7512, -8.7251) (5.7512, -8.6951) (5.751, -8.6652) (5.7507, -8.6353) (5.7502, -8.6055) (5.7495, -8.5758) (5.7487, -8.5461) (5.7478, -8.5165) (5.7467, -8.4869) (5.7454, -8.4574) (5.7439, -8.428) (5.7423, -8.3986) (5.7406, -8.3693) (5.7387, -8.34) (5.7366, -8.3109) (5.7343, -8.2817) (5.7319, -8.2527) (5.7293, -8.2237) (5.7266, -8.1948) (5.7237, -8.166) (5.7206, -8.1372) (5.7174, -8.1086) (5.714, -8.0799) (5.7104, -8.0514) (5.7067, -8.023) (5.7027, -7.9946) (5.6987, -7.9663) (5.6944, -7.9381) (5.69, -7.91) (5.6854, -7.8819) (5.6806, -7.854) (5.6756, -7.8261) (5.6705, -7.7983) (5.6652, -7.7706) (5.6597, -7.743) (5.654, -7.7156) (5.6482, -7.6882) (5.6421, -7.6609) (5.6359, -7.6337) (5.6295, -7.6066) (5.6228, -7.5796) (5.616, -7.5527) (5.609, -7.5259) (5.6019, -7.4993) (5.5945, -7.4727) (5.5869, -7.4463) (5.5791, -7.42) (5.5711, -7.3938) (5.5629, -7.3677) (5.5544, -7.3418) (5.5457, -7.316) (5.5368, -7.2904) (5.5277, -7.2649) (5.5184, -7.2395) (5.5089, -7.2142) (5.4992, -7.1891) (5.4892, -7.1642) (5.4788, -7.1395) (5.4681, -7.115) (5.4571, -7.0908) (5.4457, -7.0667) (5.4342, -7.0428) (5.4224, -7.0191) (5.4105, -6.9954) (5.3984, -6.972) (5.3859, -6.9488) (5.3726, -6.9261) (5.3612, -6.9086) (5.3521, -6.8957) (5.3458, -6.8874) (5.3426, -6.8832) knots -1 -1 -1 -1 -1 -1 -0.98571429 -0.97142857 -0.95714286 -0.94285714 -0.92857143 -0.91428571 -0.9 -0.88571429 -0.87142857 -0.85714286 -0.84285714 -0.82857143 -0.81428571 -0.8 -0.78571429 -0.77142857 -0.75714286 -0.74285714 -0.72857143 -0.71428571 -0.7 -0.68571429 -0.67142857 -0.65714286 -0.64285714 -0.62857143 -0.61428571 -0.6 -0.58571429 -0.57142857 -0.55714286 -0.54285714 -0.52857143 -0.51428571 -0.5 -0.48571429 -0.47142857 -0.45714286 -0.44285714 -0.42857143 -0.41428571 -0.4 -0.38571429 -0.37142857 -0.35714286 -0.34285714 -0.32857143 -0.31428571 -0.3 -0.28571429 -0.27142857 -0.25714286 -0.24285714 -0.22857143 -0.21428571 -0.2 -0.18571429 -0.17142857 -0.15714286 -0.14285714 -0.12857143 -0.11428571 -0.1 -0.08571429 -0.07142857 -0.05714286 -0.04285714 -0.02857143 -0.01428571 0 0 0 0 0 0
  line L9 (5.3426, -6.8832) -> (4.7509, -6.121)
  arc A18 (4.8145, -5.44) -> (4.7509, -6.121) centre (5.1459, -5.8144) ccw
  arc A19 (4.8145, -5.44) -> (5.44, -4.8145) centre (0, 0) ccw
  arc A20 (6.121, -4.7509) -> (5.44, -4.8145) centre (5.8144, -5.1459) ccw
  line L10 (6.121, -4.7509) -> (6.8832, -5.3426)
  spline S10 degree 5 poles (6.8832, -5.3426) (6.8874, -5.3458) (6.8957, -5.3521) (6.9086, -5.3612) (6.9261, -5.3726) (6.9488, -5.3859) (6.972, -5.3984) (6.9954, -5.4105) (7.0191, -5.4224) (7.0428, -5.4342) (7.0667, -5.4457) (7.0908, -5.4571) (7.115, -5.4681) (7.1395, -5.4788) (7.1642, -5.4892) (7.1891, -5.4992) (7.2142, -5.5089) (7.2395, -5.5184) (7.2649, -5.5277) (7.2904, -5.5368) (7.316, -5.5457) (7.3418, -5.5544) (7.3677, -5.5629) (7.3938, -5.5711) (7.42, -5.5791) (7.4463, -5.5869) (7.4727, -5.5945) (7.4993, -5.6019) (7.5259, -5.609) (7.5527, -5.616) (7.5796, -5.6228) (7.6066, -5.6295) (7.6337, -5.6359) (7.6609, -5.6421) (7.6882, -5.6482) (7.7156, -5.654) (7.743, -5.6597) (7.7706, -5.6652) (7.7983, -5.6705) (7.8261, -5.6756) (7.854, -5.6806) (7.8819, -5.6854) (7.91, -5.69) (7.9381, -5.6944) (7.9663, -5.6987) (7.9946, -5.7027) (8.023, -5.7067) (8.0514, -5.7104) (8.0799, -5.714) (8.1086, -5.7174) (8.1372, -5.7206) (8.166, -5.7237) (8.1948, -5.7266) (8.2237, -5.7293) (8.2527, -5.7319) (8.2817, -5.7343) (8.3109, -5.7366) (8.34, -5.7387) (8.3693, -5.7406) (8.3986, -5.7423) (8.428, -5.7439) (8.4574, -5.7454) (8.4869, -5.7467) (8.5165, -5.7478) (8.5461, -5.7487) (8.5758, -5.7495) (8.6055, -5.7502) (8.6353, -5.7507) (8.6652, -5.751) (8.6951, -5.7512) (8.7251, -5.7512) (8.7491, -5.7511) (8.7671, -5.7509) (8.7791, -5.7508) (8.7852, -5.7507) knots 0 0 0 0 0 0 0.01428571 0.02857143 0.04285714 0.05714286 0.07142857 0.08571429 0.1 0.11428571 0.12857143 0.14285714 0.15714286 0.17142857 0.18571429 0.2 0.21428571 0.22857143 0.24285714 0.25714286 0.27142857 0.28571429 0.3 0.31428571 0.32857143 0.34285714 0.35714286 0.37142857 0.38571429 0.4 0.41428571 0.42857143 0.44285714 0.45714286 0.47142857 0.48571429 0.5 0.51428571 0.52857143 0.54285714 0.55714286 0.57142857 0.58571429 0.6 0.61428571 0.62857143 0.64285714 0.65714286 0.67142857 0.68571429 0.7 0.71428571 0.72857143 0.74285714 0.75714286 0.77142857 0.78571429 0.8 0.81428571 0.82857143 0.84285714 0.85714286 0.87142857 0.88571429 0.9 0.91428571 0.92857143 0.94285714 0.95714286 0.97142857 0.98571429 1 1 1 1 1 1
  arc A21 (8.7852, -5.7507) -> (9.3729, -4.7328) centre (0, 0) ccw
  spline S11 degree 5 poles (9.3729, -4.7328) (9.3699, -4.7276) (9.364, -4.7171) (9.3551, -4.7014) (9.3432, -4.6805) (9.3282, -4.6546) (9.3131, -4.6288) (9.2979, -4.6031) (9.2826, -4.5775) (9.2671, -4.5521) (9.2516, -4.5268) (9.236, -4.5016) (9.2202, -4.4766) (9.2044, -4.4516) (9.1884, -4.4269) (9.1723, -4.4022) (9.1561, -4.3777) (9.1398, -4.3534) (9.1234, -4.3291) (9.1069, -4.305) (9.0903, -4.2811) (9.0736, -4.2573) (9.0568, -4.2336) (9.0399, -4.2101) (9.0228, -4.1867) (9.0057, -4.1635) (8.9884, -4.1404) (8.9711, -4.1175) (8.9536, -4.0948) (8.936, -4.0721) (8.9183, -4.0497) (8.9005, -4.0274) (8.8826, -4.0052) (8.8646, -3.9833) (8.8465, -3.9614) (8.8283, -3.9398) (8.8099, -3.9183) (8.7915, -3.897) (8.773, -3.8758) (8.7543, -3.8549) (8.7355, -3.8341) (8.7166, -3.8134) (8.6976, -3.793) (8.6785, -3.7728) (8.6593, -3.7527) (8.64, -3.7328) (8.6205, -3.7131) (8.601, -3.6936) (8.5813, -3.6743) (8.5615, -3.6552) (8.5416, -3.6363) (8.5216, -3.6176) (8.5014, -3.5992) (8.4812, -3.581) (8.4608, -3.563) (8.4402, -3.5453) (8.4196, -3.5277) (8.3989, -3.5104) (8.378, -3.4932) (8.357, -3.4764) (8.3359, -3.4598) (8.3146, -3.4436) (8.293, -3.4277) (8.2714, -3.4122) (8.2495, -3.3971) (8.2275, -3.3822) (8.2055, -3.3675) (8.1834, -3.3529) (8.1611, -3.3387) (8.1387, -3.3249) (8.1159, -3.3119) (8.0972, -3.3024) (8.0829, -3.2958) (8.0733, -3.2917) (8.0684, -3.2898) knots -1 -1 -1 -1 -1 -1 -0.98571429 -0.97142857 -0.95714286 -0.94285714 -0.92857143 -0.91428571 -0.9 -0.88571429 -0.87142857 -0.85714286 -0.84285714 -0.82857143 -0.81428571 -0.8 -0.78571429 -0.77142857 -0.75714286 -0.74285714 -0.72857143 -0.71428571 -0.7 -0.68571429 -0.67142857 -0.65714286 -0.64285714 -0.62857143 -0.61428571 -0.6 -0.58571429 -0.57142857 -0.55714286 -0.54285714 -0.52857143 -0.51428571 -0.5 -0.48571429 -0.47142857 -0.45714286 -0.44285714 -0.42857143 -0.41428571 -0.4 -0.38571429 -0.37142857 -0.35714286 -0.34285714 -0.32857143 -0.31428571 -0.3 -0.28571429 -0.27142857 -0.25714286 -0.24285714 -0.22857143 -0.21428571 -0.2 -0.18571429 -0.17142857 -0.15714286 -0.14285714 -0.12857143 -0.11428571 -0.1 -0.08571429 -0.07142857 -0.05714286 -0.04285714 -0.02857143 -0.01428571 0 0 0 0 0 0
  line L11 (8.0684, -3.2898) -> (7.1749, -2.9254)
  arc A22 (6.8895, -2.3039) -> (7.1749, -2.9254) centre (7.3637, -2.4624) ccw
  arc A23 (6.8895, -2.3039) -> (7.1184, -1.4495) centre (0, 0) ccw
  arc A24 (7.6764, -1.0539) -> (7.1184, -1.4495) centre (7.6084, -1.5493) ccw
  line L12 (7.6764, -1.0539) -> (8.6323, -1.1852)
  spline S12 degree 5 poles (8.6323, -1.1852) (8.6375, -1.1859) (8.6479, -1.1872) (8.6636, -1.1886) (8.6845, -1.1897) (8.7108, -1.1899) (8.7371, -1.1892) (8.7635, -1.188) (8.7899, -1.1864) (8.8164, -1.1847) (8.8428, -1.1828) (8.8693, -1.1806) (8.8958, -1.178) (8.9224, -1.1751) (8.949, -1.1717) (8.9756, -1.1679) (9.0022, -1.1638) (9.0288, -1.1594) (9.0554, -1.1547) (9.0821, -1.1498) (9.1087, -1.1447) (9.1354, -1.1393) (9.1621, -1.1337) (9.1887, -1.1278) (9.2154, -1.1217) (9.2421, -1.1153) (9.2688, -1.1086) (9.2955, -1.1017) (9.3222, -1.0946) (9.3488, -1.0873) (9.3755, -1.0797) (9.4022, -1.072) (9.4289, -1.064) (9.4555, -1.0558) (9.4822, -1.0474) (9.5089, -1.0387) (9.5355, -1.0299) (9.5622, -1.0209) (9.5888, -1.0116) (9.6154, -1.0022) (9.642, -0.9925) (9.6686, -0.9827) (9.6952, -0.9727) (9.7218, -0.9624) (9.7483, -0.952) (9.7749, -0.9414) (9.8014, -0.9306) (9.8279, -0.9196) (9.8544, -0.9085) (9.8809, -0.8971) (9.9074, -0.8856) (9.9338, -0.8739) (9.9602, -0.862) (9.9866, -0.8499) (10.013, -0.8376) (10.0394, -0.8252) (10.0657, -0.8126) (10.092, -0.7998) (10.1183, -0.7868) (10.1446, -0.7737) (10.1708, -0.7604) (10.197, -0.7469) (10.2232, -0.7333) (10.2494, -0.7195) (10.2755, -0.7055) (10.3016, -0.6914) (10.3277, -0.677) (10.3538, -0.6626) (10.3798, -0.6479) (10.4058, -0.6331) (10.4317, -0.6182) (10.4525, -0.6061) (10.468, -0.5969) (10.4784, -0.5908) (10.4835, -0.5877) knots 0 0 0 0 0 0 0.01428571 0.02857143 0.04285714 0.05714286 0.07142857 0.08571429 0.1 0.11428571 0.12857143 0.14285714 0.15714286 0.17142857 0.18571429 0.2 0.21428571 0.22857143 0.24285714 0.25714286 0.27142857 0.28571429 0.3 0.31428571 0.32857143 0.34285714 0.35714286 0.37142857 0.38571429 0.4 0.41428571 0.42857143 0.44285714 0.45714286 0.47142857 0.48571429 0.5 0.51428571 0.52857143 0.54285714 0.55714286 0.57142857 0.58571429 0.6 0.61428571 0.62857143 0.64285714 0.65714286 0.67142857 0.68571429 0.7 0.71428571 0.72857143 0.74285714 0.75714286 0.77142857 0.78571429 0.8 0.81428571 0.82857143 0.84285714 0.85714286 0.87142857 0.88571429 0.9 0.91428571 0.92857143 0.94285714 0.95714286 0.97142857 0.98571429 1 1 1 1 1 1
  arc A25 (10.4835, -0.5877) -> (10.4835, 0.5877) centre (0, 0) ccw
  spline S13 degree 5 poles (10.4835, 0.5877) (10.4784, 0.5908) (10.468, 0.5969) (10.4525, 0.6061) (10.4317, 0.6182) (10.4058, 0.6331) (10.3798, 0.6479) (10.3538, 0.6626) (10.3277, 0.677) (10.3016, 0.6914) (10.2755, 0.7055) (10.2494, 0.7195) (10.2232, 0.7333) (10.197, 0.7469) (10.1708, 0.7604) (10.1446, 0.7737) (10.1183, 0.7868) (10.092, 0.7998) (10.0657, 0.8126) (10.0394, 0.8252) (10.013, 0.8376) (9.9866, 0.8499) (9.9602, 0.862) (9.9338, 0.8739) (9.9074, 0.8856) (9.8809, 0.8971) (9.8544, 0.9085) (9.8279, 0.9196) (9.8014, 0.9306) (9.7749, 0.9414) (9.7483, 0.952) (9.7218, 0.9624) (9.6952, 0.9727) (9.6686, 0.9827) (9.642, 0.9925) (9.6154, 1.0022) (9.5888, 1.0116) (9.5622, 1.0209) (9.5355, 1.0299) (9.5089, 1.0387) (9.4822, 1.0474) (9.4555, 1.0558) (9.4289, 1.064) (9.4022, 1.072) (9.3755, 1.0797) (9.3488, 1.0873) (9.3222, 1.0946) (9.2955, 1.1017) (9.2688, 1.1086) (9.2421, 1.1153) (9.2154, 1.1217) (9.1887, 1.1278) (9.1621, 1.1337) (9.1354, 1.1393) (9.1087, 1.1447) (9.0821, 1.1498) (9.0554, 1.1547) (9.0288, 1.1594) (9.0022, 1.1638) (8.9756, 1.1679) (8.949, 1.1717) (8.9224, 1.1751) (8.8958, 1.178) (8.8693, 1.1806) (8.8428, 1.1828) (8.8164, 1.1847) (8.7899, 1.1864) (8.7635, 1.188) (8.7371, 1.1892) (8.7108, 1.1899) (8.6845, 1.1897) (8.6636, 1.1886) (8.6479, 1.1872) (8.6375, 1.1859) (8.6323, 1.1852) knots -1 -1 -1 -1 -1 -1 -0.98571429 -0.97142857 -0.95714286 -0.94285714 -0.92857143 -0.91428571 -0.9 -0.88571429 -0.87142857 -0.85714286 -0.84285714 -0.82857143 -0.81428571 -0.8 -0.78571429 -0.77142857 -0.75714286 -0.74285714 -0.72857143 -0.71428571 -0.7 -0.68571429 -0.67142857 -0.65714286 -0.64285714 -0.62857143 -0.61428571 -0.6 -0.58571429 -0.57142857 -0.55714286 -0.54285714 -0.52857143 -0.51428571 -0.5 -0.48571429 -0.47142857 -0.45714286 -0.44285714 -0.42857143 -0.41428571 -0.4 -0.38571429 -0.37142857 -0.35714286 -0.34285714 -0.32857143 -0.31428571 -0.3 -0.28571429 -0.27142857 -0.25714286 -0.24285714 -0.22857143 -0.21428571 -0.2 -0.18571429 -0.17142857 -0.15714286 -0.14285714 -0.12857143 -0.11428571 -0.1 -0.08571429 -0.07142857 -0.05714286 -0.04285714 -0.02857143 -0.01428571 0 0 0 0 0 0
  line L13 (8.6323, 1.1852) -> (7.6764, 1.0539)
  arc A26 (7.1184, 1.4495) -> (7.6764, 1.0539) centre (7.6084, 1.5493) ccw
  arc A27 (7.1184, 1.4495) -> (6.8895, 2.3039) centre (0, 0) ccw
  arc A28 (7.1749, 2.9254) -> (6.8895, 2.3039) centre (7.3637, 2.4624) ccw
  line L14 (7.1749, 2.9254) -> (8.0684, 3.2898)
  spline S14 degree 5 poles (8.0684, 3.2898) (8.0733, 3.2917) (8.0829, 3.2958) (8.0972, 3.3024) (8.1159, 3.3119) (8.1387, 3.3249) (8.1611, 3.3387) (8.1834, 3.3529) (8.2055, 3.3675) (8.2275, 3.3822) (8.2495, 3.3971) (8.2714, 3.4122) (8.293, 3.4277) (8.3146, 3.4436) (8.3359, 3.4598) (8.357, 3.4764) (8.378, 3.4932) (8.3989, 3.5104) (8.4196, 3.5277) (8.4402, 3.5453) (8.4608, 3.563) (8.4812, 3.581) (8.5014, 3.5992) (8.5216, 3.6176) (8.5416, 3.6363) (8.5615, 3.6552) (8.5813, 3.6743) (8.601, 3.6936) (8.6205, 3.7131) (8.64, 3.7328) (8.6593, 3.7527) (8.6785, 3.7728) (8.6976, 3.793) (8.7166, 3.8134) (8.7355, 3.8341) (8.7543, 3.8549) (8.773, 3.8758) (8.7915, 3.897) (8.8099, 3.9183) (8.8283, 3.9398) (8.8465, 3.9614) (8.8646, 3.9833) (8.8826, 4.0052) (8.9005, 4.0274) (8.9183, 4.0497) (8.936, 4.0721) (8.9536, 4.0948) (8.9711, 4.1175) (8.9884, 4.1404) (9.0057, 4.1635) (9.0228, 4.1867) (9.0399, 4.2101) (9.0568, 4.2336) (9.0736, 4.2573) (9.0903, 4.2811) (9.1069, 4.305) (9.1234, 4.3291) (9.1398, 4.3534) (9.1561, 4.3777) (9.1723, 4.4022) (9.1884, 4.4269) (9.2044, 4.4516) (9.2202, 4.4766) (9.236, 4.5016) (9.2516, 4.5268) (9.2671, 4.5521) (9.2826, 4.5775) (9.2979, 4.6031) (9.3131, 4.6288) (9.3282, 4.6546) (9.3432, 4.6805) (9.3551, 4.7014) (9.364, 4.7171) (9.3699, 4.7276) (9.3729, 4.7328) knots 0 0 0 0 0 0 0.01428571 0.02857143 0.04285714 0.05714286 0.07142857 0.08571429 0.1 0.11428571 0.12857143 0.14285714 0.15714286 0.17142857 0.18571429 0.2 0.21428571 0.22857143 0.24285714 0.25714286 0.27142857 0.28571429 0.3 0.31428571 0.32857143 0.34285714 0.35714286 0.37142857 0.38571429 0.4 0.41428571 0.42857143 0.44285714 0.45714286 0.47142857 0.48571429 0.5 0.51428571 0.52857143 0.54285714 0.55714286 0.57142857 0.58571429 0.6 0.61428571 0.62857143 0.64285714 0.65714286 0.67142857 0.68571429 0.7 0.71428571 0.72857143 0.74285714 0.75714286 0.77142857 0.78571429 0.8 0.81428571 0.82857143 0.84285714 0.85714286 0.87142857 0.88571429 0.9 0.91428571 0.92857143 0.94285714 0.95714286 0.97142857 0.98571429 1 1 1 1 1 1
  arc A29 (9.3729, 4.7328) -> (8.7852, 5.7507) centre (0, 0) ccw
  spline S15 degree 5 poles (8.7852, 5.7507) (8.7791, 5.7508) (8.7671, 5.7509) (8.7491, 5.7511) (8.7251, 5.7512) (8.6951, 5.7512) (8.6652, 5.751) (8.6353, 5.7507) (8.6055, 5.7502) (8.5758, 5.7495) (8.5461, 5.7487) (8.5165, 5.7478) (8.4869, 5.7467) (8.4574, 5.7454) (8.428, 5.7439) (8.3986, 5.7423) (8.3693, 5.7406) (8.34, 5.7387) (8.3109, 5.7366) (8.2817, 5.7343) (8.2527, 5.7319) (8.2237, 5.7293) (8.1948, 5.7266) (8.166, 5.7237) (8.1372, 5.7206) (8.1086, 5.7174) (8.0799, 5.714) (8.0514, 5.7104) (8.023, 5.7067) (7.9946, 5.7027) (7.9663, 5.6987) (7.9381, 5.6944) (7.91, 5.69) (7.8819, 5.6854) (7.854, 5.6806) (7.8261, 5.6756) (7.7983, 5.6705) (7.7706, 5.6652) (7.743, 5.6597) (7.7156, 5.654) (7.6882, 5.6482) (7.6609, 5.6421) (7.6337, 5.6359) (7.6066, 5.6295) (7.5796, 5.6228) (7.5527, 5.616) (7.5259, 5.609) (7.4993, 5.6019) (7.4727, 5.5945) (7.4463, 5.5869) (7.42, 5.5791) (7.3938, 5.5711) (7.3677, 5.5629) (7.3418, 5.5544) (7.316, 5.5457) (7.2904, 5.5368) (7.2649, 5.5277) (7.2395, 5.5184) (7.2142, 5.5089) (7.1891, 5.4992) (7.1642, 5.4892) (7.1395, 5.4788) (7.115, 5.4681) (7.0908, 5.4571) (7.0667, 5.4457) (7.0428, 5.4342) (7.0191, 5.4224) (6.9954, 5.4105) (6.972, 5.3984) (6.9488, 5.3859) (6.9261, 5.3726) (6.9086, 5.3612) (6.8957, 5.3521) (6.8874, 5.3458) (6.8832, 5.3426) knots -1 -1 -1 -1 -1 -1 -0.98571429 -0.97142857 -0.95714286 -0.94285714 -0.92857143 -0.91428571 -0.9 -0.88571429 -0.87142857 -0.85714286 -0.84285714 -0.82857143 -0.81428571 -0.8 -0.78571429 -0.77142857 -0.75714286 -0.74285714 -0.72857143 -0.71428571 -0.7 -0.68571429 -0.67142857 -0.65714286 -0.64285714 -0.62857143 -0.61428571 -0.6 -0.58571429 -0.57142857 -0.55714286 -0.54285714 -0.52857143 -0.51428571 -0.5 -0.48571429 -0.47142857 -0.45714286 -0.44285714 -0.42857143 -0.41428571 -0.4 -0.38571429 -0.37142857 -0.35714286 -0.34285714 -0.32857143 -0.31428571 -0.3 -0.28571429 -0.27142857 -0.25714286 -0.24285714 -0.22857143 -0.21428571 -0.2 -0.18571429 -0.17142857 -0.15714286 -0.14285714 -0.12857143 -0.11428571 -0.1 -0.08571429 -0.07142857 -0.05714286 -0.04285714 -0.02857143 -0.01428571 0 0 0 0 0 0
  line L15 (6.8832, 5.3426) -> (6.121, 4.7509)
  arc A30 (5.44, 4.8145) -> (6.121, 4.7509) centre (5.8144, 5.1459) ccw
  arc A31 (5.44, 4.8145) -> (4.8145, 5.44) centre (0, 0) ccw
  arc A32 (4.7509, 6.121) -> (4.8145, 5.44) centre (5.1459, 5.8144) ccw
  line L16 (4.7509, 6.121) -> (5.3426, 6.8832)
  spline S16 degree 5 poles (5.3426, 6.8832) (5.3458, 6.8874) (5.3521, 6.8957) (5.3612, 6.9086) (5.3726, 6.9261) (5.3859, 6.9488) (5.3984, 6.972) (5.4105, 6.9954) (5.4224, 7.0191) (5.4342, 7.0428) (5.4457, 7.0667) (5.4571, 7.0908) (5.4681, 7.115) (5.4788, 7.1395) (5.4892, 7.1642) (5.4992, 7.1891) (5.5089, 7.2142) (5.5184, 7.2395) (5.5277, 7.2649) (5.5368, 7.2904) (5.5457, 7.316) (5.5544, 7.3418) (5.5629, 7.3677) (5.5711, 7.3938) (5.5791, 7.42) (5.5869, 7.4463) (5.5945, 7.4727) (5.6019, 7.4993) (5.609, 7.5259) (5.616, 7.5527) (5.6228, 7.5796) (5.6295, 7.6066) (5.6359, 7.6337) (5.6421, 7.6609) (5.6482, 7.6882) (5.654, 7.7156) (5.6597, 7.743) (5.6652, 7.7706) (5.6705, 7.7983) (5.6756, 7.8261) (5.6806, 7.854) (5.6854, 7.8819) (5.69, 7.91) (5.6944, 7.9381) (5.6987, 7.9663) (5.7027, 7.9946) (5.7067, 8.023) (5.7104, 8.0514) (5.714, 8.0799) (5.7174, 8.1086) (5.7206, 8.1372) (5.7237, 8.166) (5.7266, 8.1948) (5.7293, 8.2237) (5.7319, 8.2527) (5.7343, 8.2817) (5.7366, 8.3109) (5.7387, 8.34) (5.7406, 8.3693) (5.7423, 8.3986) (5.7439, 8.428) (5.7454, 8.4574) (5.7467, 8.4869) (5.7478, 8.5165) (5.7487, 8.5461) (5.7495, 8.5758) (5.7502, 8.6055) (5.7507, 8.6353) (5.751, 8.6652) (5.7512, 8.6951) (5.7512, 8.7251) (5.7511, 8.7491) (5.7509, 8.7671) (5.7508, 8.7791) (5.7507, 8.7852) knots 0 0 0 0 0 0 0.01428571 0.02857143 0.04285714 0.05714286 0.07142857 0.08571429 0.1 0.11428571 0.12857143 0.14285714 0.15714286 0.17142857 0.18571429 0.2 0.21428571 0.22857143 0.24285714 0.25714286 0.27142857 0.28571429 0.3 0.31428571 0.32857143 0.34285714 0.35714286 0.37142857 0.38571429 0.4 0.41428571 0.42857143 0.44285714 0.45714286 0.47142857 0.48571429 0.5 0.51428571 0.52857143 0.54285714 0.55714286 0.57142857 0.58571429 0.6 0.61428571 0.62857143 0.64285714 0.65714286 0.67142857 0.68571429 0.7 0.71428571 0.72857143 0.74285714 0.75714286 0.77142857 0.78571429 0.8 0.81428571 0.82857143 0.84285714 0.85714286 0.87142857 0.88571429 0.9 0.91428571 0.92857143 0.94285714 0.95714286 0.97142857 0.98571429 1 1 1 1 1 1
  arc A33 (5.7507, 8.7852) -> (4.7328, 9.3729) centre (0, 0) ccw